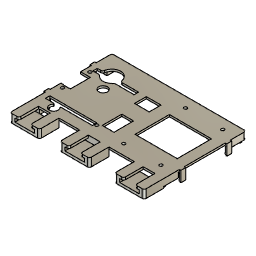
nextion_display_obd_holder_FUSION360 (Autodesk Fusion 360 design; units mm, degrees)
Autodesk Fusion 360 part; units mm, degrees
sketch "Sketch1" plane through (0, 0, 0) normal (0, 0, 1) x (1, 0, 0)
  line L0 (68.45, -42) -> (-68.45, -42)
  line L1 (-68.45, -42) -> (-68.45, 42)
  line L2 (-68.45, 42) -> (68.45, 42)
  line L3 (68.45, 42) -> (68.45, -42)
  line L4 (68.45, -42) -> (-68.45, 42) construction
  line L5 (-68.45, -42) -> (68.45, 42) construction
  line L6 (65.25, -38.9) -> (-65.25, -38.9) construction
  line L7 (-65.25, -38.9) -> (-65.25, 38.9) construction
  line L8 (-65.25, 38.9) -> (65.25, 38.9) construction
  line L9 (65.25, 38.9) -> (65.25, -38.9) construction
  line L10 (65.25, -38.9) -> (-65.25, 38.9) construction
  line L11 (-65.25, -38.9) -> (65.25, 38.9) construction
  circle A0 centre (-65.25, 38.9) radius 1.45
  circle A1 centre (65.25, 38.9) radius 1.45
  circle A2 centre (65.25, -38.9) radius 1.45
  circle A3 centre (-65.25, -38.9) radius 1.45
  line L12 (-68.45, 42) -> (-58.45, 42)
  line L13 (-58.45, 42) -> (-58.45, 27)
  line L14 (-58.45, 27) -> (-68.45, 27)
  line L15 (-68.45, 27) -> (-68.45, 42)
  line L16 (-68.45, -42) -> (-58.45, -42)
  line L17 (-58.45, -42) -> (-58.45, -27)
  line L18 (-58.45, -27) -> (-68.45, -27)
  line L19 (68.45, 42) -> (58.45, 42)
  line L20 (58.45, 42) -> (58.45, 27)
  line L21 (58.45, 27) -> (68.45, 27)
  line L22 (68.45, 27) -> (68.45, 42)
  line L23 (68.45, -42) -> (58.45, -42)
  line L24 (58.45, -42) -> (58.45, -27)
  line L25 (58.45, -27) -> (68.45, -27)
  line L26 (68.45, -27) -> (68.45, -42)
  line L27 (25, -30) -> (-25, -30)
  line L28 (-25, -30) -> (-25, 30)
  line L29 (-25, 30) -> (25, 30)
  line L30 (25, 30) -> (25, -30)
  line L31 (25, -30) -> (-25, 30) construction
  line L32 (-25, -30) -> (25, 30) construction
  line L33 (-58.45, -10) -> (-68.45, -10)
  line L34 (-68.45, -10) -> (-68.45, 10)
  line L35 (-68.45, 10) -> (-58.45, 10)
  line L36 (-58.45, 10) -> (-58.45, -10)
  line L37 (-58.45, -10) -> (-68.45, 10) construction
  line L38 (-68.45, -10) -> (-58.45, 10) construction
  line L39 (-12.45, -35) -> (7.55, -35)
  line L40 (7.55, -35) -> (7.55, -42)
  line L41 (7.55, -42) -> (-12.45, -42)
  line L42 (-12.45, -42) -> (-12.45, -35)
  circle A4 centre (-48.45, 22) radius 9
  circle A5 centre (-50.45, -35.5) radius 4.5
  circle A6 centre (-41.45, 6) radius 4.5
  line L43 (68.45, -21) -> (69.95, -21)
  line L44 (69.95, -21) -> (69.95, -26)
  line L45 (69.95, -26) -> (68.45, -26)
  line L46 (68.45, -26) -> (68.45, -21)
  point P0 (-63.45, 0)
  dimension "d1" = 136.9
  dimension "d2" = 84
  dimension "d3" = 130.5
  dimension "d4" = 77.8
  dimension "d5" = 2.9
  dimension "d6" = 2.9
  dimension "d7" = 2.9
  dimension "d8" = 2.9
  dimension "d9" = 10
  dimension "d10" = 15
  dimension "d11" = 10
  dimension "d12" = 15
  dimension "d13" = 10
  dimension "d14" = 15
  dimension "d15" = 10
  dimension "d16" = 15
  dimension "d25" = 50
  dimension "d26" = 60
  dimension "d60" = 10
  dimension "d61" = 20
  dimension "d62" = 20
  dimension "d63" = 7
  dimension "d64" = 18
  dimension "d65" = 20
  dimension "d66" = 20
  dimension "d67" = 9
  dimension "d68" = 18
  dimension "d69" = 6.5
  dimension "d70" = 9
  dimension "d71" = 27
  dimension "d72" = 36
  dimension "d134" = 56
  dimension "d148" = 1.5
  dimension "d149" = 5
  dimension "d150" = 1
  constraint horizontal L0
  constraint perpendicular L0 L1
  constraint parallel L0 L2
  constraint parallel L1 L3
  constraint coincident L4 origin
  constraint coincident L5 origin
  constraint horizontal L6
  constraint perpendicular L6 L7
  constraint parallel L6 L8
  constraint parallel L7 L9
  constraint coincident L10 origin
  constraint coincident L11 origin
  constraint coincident L7.end L8.start
  constraint coincident L8.end L9.start
  constraint coincident L6.start L9.end
  constraint coincident L6.end L7.start
  constraint horizontal L12
  constraint vertical L13
  constraint horizontal L14
  constraint vertical L15
  constraint horizontal L16
  constraint vertical L17
  constraint horizontal L18
  constraint horizontal L19
  constraint vertical L20
  constraint horizontal L21
  constraint vertical L22
  constraint horizontal L23
  constraint vertical L24
  constraint horizontal L25
  constraint vertical L26
  constraint horizontal L27
  constraint perpendicular L27 L28
  constraint parallel L27 L29
  constraint parallel L28 L30
  constraint coincident L31 origin
  constraint coincident L32 origin
  constraint horizontal L33
  constraint perpendicular L33 L34
  constraint parallel L33 L35
  constraint parallel L34 L36
  constraint coincident L37 P0
  constraint coincident L38 P0
  constraint midpoint L1 L34
  constraint horizontal L39
  constraint vertical L40
  constraint horizontal L41
  constraint vertical L42
  constraint horizontal L43
  constraint vertical L44
  constraint horizontal L45
  constraint vertical L46
  constraint coincident L3 L43.start
  measures "d1" distance of L1.end L2.end
  measures "d2" distance of L0.end L1.end
  measures "d3" distance of L7.end L8.end
  measures "d4" distance of L6.end L7.end
  measures "d5" diameter of A0
  measures "d6" diameter of A1
  measures "d7" diameter of A2
  measures "d8" diameter of A3
  measures "d9" distance of L1.end L12.end
  measures "d10" distance of L1.end L14.end
  measures "d11" distance of L0.end L16.end
  measures "d12" distance of L0.end L18.end
  measures "d13" distance of L2.end L19.end
  measures "d14" distance of L2.end L21.end
  measures "d15" distance of L0.start L23.end
  measures "d16" distance of L0.start L25.end
  measures "d25" distance of L28.end L29.end
  measures "d26" distance of L27.end L28.end
  measures "d60" distance of L34.end L35.end
  measures "d61" distance of L33.end L34.end
  measures "d62" distance of L39.start L39.end
  measures "d63" distance of L39.start L41.end
  measures "d64" diameter of A4
  measures "d65" distance of L2 A4.centre
  measures "d66" distance of L1 A4.centre
  measures "d67" diameter of A5
  measures "d68" distance of L1 A5.centre
  measures "d69" distance of L0 A5.centre
  measures "d70" diameter of A6
  measures "d71" distance of L1 A6.centre
  measures "d72" distance of L2 A6.centre
  measures "d134" distance of L1 L42
  measures "d148" distance of L43.start L43.end
  measures "d149" distance of L43.start L45.end
  measures "d150" distance of L25 L45
extrude "Extrude1" add sketch "Sketch1" along normal blind 2 contours L0 L3 L23 L24 L25 L26 | L0 L1 L2 L3 L13 L14 L17 L18 L20 L21 L24 L25 L33 L35 L36 L39 L40 L42 L46 | L0 L39 L40 L41 L42 | L0 L1 L16 L17 L18 | L2 L3 L19 L20 L21 L22 | L1 L2 L12 L13 L14 L15 | A0 | A1 | A2 | A3 | L27 L28 L29 L30 makes body 1
extrude "Extrude2" add sketch "Sketch1" against normal blind 5 contours L0 L3 L23 L24 L25 L26 | L0 L39 L40 L41 L42 | L0 L1 L16 L17 L18 | L2 L3 L19 L20 L21 L22 | L1 L2 L12 L13 L14 L15 bodies 1
extrude "Extrude3" add sketch "Sketch1" against normal blind 8 contours A0 | A1 | A2 | A3 bodies 1
chamfer "Chamfer1" distance 0.5 angle 45 4 edges at (63.8981, 39.4243, -8) (63.8981, -38.3757, -8) (-66.6019, -38.3757, -8) (-66.6019, 39.4243, -8) on bodies 1
fillet "Fillet2" radius 2 2 edges at (-68.45, 42, -1.5) (68.45, 42, -1.5) on bodies 1
sketch "Sketch6" plane through (0, 0, 2) normal (0, 0, 1) x (-1, 0, 0)
  arc A0 (-68.45, -40) -> (-66.45, -42) centre (-66.45, -40) ccw
  line L0 (-66.45, -42) -> (66.45, -42)
  arc A1 (66.45, -42) -> (68.45, -40) centre (66.45, -40) ccw
  line L1 (68.45, -40) -> (68.45, -10)
  line L2 (68.45, -10) -> (58.45, -10)
  line L3 (58.45, -10) -> (58.45, 10)
  line L4 (58.45, 10) -> (68.45, 10)
  line L5 (68.45, 10) -> (68.45, 42)
  line L6 (68.45, 42) -> (-68.45, 42)
  line L7 (-68.45, 42) -> (-68.45, -40)
  circle A2 centre (48.45, -22) radius 9
  circle A3 centre (41.45, -6) radius 4.5
  circle A4 centre (50.45, 35.5) radius 4.5
  line L8 (-60.7116, 31.6265) -> (-22.7116, 31.6265)
  line L9 (-22.7116, 31.6265) -> (-22.7116, -31.3735)
  line L10 (-22.7116, -31.3735) -> (-60.7116, -31.3735)
  line L11 (-60.7116, -31.3735) -> (-60.7116, 31.6265)
  line L12 (-60.7116, 31.6265) -> (-22.7116, -31.3735) construction
  line L13 (-22.7116, 31.6265) -> (-60.7116, -31.3735) construction
  point P0 (-41.7116, 0.1265)
  dimension "d91" = 38
  dimension "d92" = 63
  constraint horizontal L8
  constraint perpendicular L8 L9
  constraint parallel L8 L10
  constraint parallel L9 L11
  constraint coincident L12 P0
  constraint coincident L13 P0
  measures "d91" distance of L9.end L10.end
  measures "d92" distance of L8.end L9.end
sketch "Sketch7" plane through (0, 0, 0) normal (0, 0, 1) x (1, 0, 0)
  line L0 (55.2284, -31.5) -> (17.2284, -31.5)
  line L1 (17.2284, -31.5) -> (17.2284, 31.5)
  line L2 (17.2284, 31.5) -> (55.2284, 31.5)
  line L3 (55.2284, 31.5) -> (55.2284, -31.5)
  line L4 (55.2284, -31.5) -> (17.2284, 31.5) construction
  line L5 (17.2284, -31.5) -> (55.2284, 31.5) construction
  line L6 (57.7284, -17.5) -> (14.7284, -17.5)
  line L7 (14.7284, -17.5) -> (14.7284, 17.5)
  line L8 (14.7284, 17.5) -> (57.7284, 17.5)
  line L9 (57.7284, 17.5) -> (57.7284, -17.5)
  line L10 (57.7284, -17.5) -> (14.7284, 17.5) construction
  line L11 (14.7284, -17.5) -> (57.7284, 17.5) construction
  point P0 (36.2284, 0)
  point P1 (36.2284, 0)
  dimension "d95" = 38
  dimension "d96" = 63
  dimension "d97" = 43
  dimension "d98" = 35
  dimension "d135" = 31.5
  constraint horizontal L0
  constraint perpendicular L0 L1
  constraint parallel L0 L2
  constraint parallel L1 L3
  constraint coincident L4 P1
  constraint coincident L5 P1
  constraint horizontal L6
  constraint perpendicular L6 L7
  constraint parallel L6 L8
  constraint parallel L7 L9
  constraint coincident L10 P1
  constraint coincident L11 P1
  constraint coincident P1 P0
  measures "d95" distance of L1.end L2.end
  measures "d96" distance of L0.end L1.end
  measures "d97" distance of L7.end L8.end
  measures "d98" distance of L6.end L7.end
  measures "d135" distance of origin L2
hole "Hole1" at (17.2284, 31.5, 0) at (55.2284, 31.5, 0) at (55.2284, -31.5, 0) at (17.2284, -31.5, 0) direction (0, 0, 1) diameter 3.2 depth 26 tip angle 180 bodies 1
extrude "Extrude8" cut sketch "Sketch7" along normal blind 19 contours L1 L3 L6 L8 | L3 L6 L8 L9 | L1 L6 L7 L8 bodies 1
sketch "Sketch8" plane through (0, 0, 0) normal (0, 0, 1) x (1, 0, 0)
  line L0 (2.0938, 21.5699) -> (-62.9062, 21.5699)
  line L1 (2.0938, 21.5699) -> (2.0938, -31.4301)
  line L2 (-62.9062, 21.5699) -> (-62.9062, 19.5699)
  line L3 (-62.9062, 19.5699) -> (-62.9062, 16.5699) construction
  line L4 (-62.9062, 16.5699) -> (-65.9062, 16.5699) construction
  line L5 (2.0938, -31.4301) -> (-62.9062, -31.4301)
  line L6 (-62.9062, -31.4301) -> (-62.9062, -18.4301)
  line L7 (-62.9062, -18.4301) -> (-62.9062, -15.4301) construction
  line L8 (-62.9062, -15.4301) -> (-65.9062, -15.4301) construction
  line L9 (-62.9062, -18.4301) -> (-65.9062, -15.4301)
  line L10 (-65.9062, -15.4301) -> (-65.9062, 16.5699)
  line L11 (-65.9062, 16.5699) -> (-62.9062, 19.5699)
  circle A0 centre (-12.9062, -28.9301) radius 1.6
  circle A1 centre (-63.4062, 14.5699) radius 1.6
  circle A2 centre (-63.4062, -13.4301) radius 1.6
  line L12 (2.0938, 21.5699) -> (-12.9062, 21.5699)
  line L13 (-12.9062, 21.5699) -> (-12.9062, 9.5699)
  line L14 (-12.9062, 9.5699) -> (2.0938, 9.5699)
  line L15 (2.0938, 9.5699) -> (2.0938, 21.5699)
  line L16 (2.0938, -6.4301) -> (-9.9062, -6.4301)
  line L17 (-9.9062, -6.4301) -> (-9.9062, -26.4301)
  line L18 (-9.9062, -26.4301) -> (2.0938, -26.4301)
  line L19 (2.0938, -26.4301) -> (2.0938, -6.4301)
  line L20 (-62.9062, 21.5699) -> (-20.9062, 21.5699)
  line L21 (-20.9062, 21.5699) -> (-20.9062, 17.0699)
  line L22 (-20.9062, 17.0699) -> (-62.9062, 17.0699)
  line L23 (-62.9062, 17.0699) -> (-62.9062, 21.5699)
  line L24 (-62.9062, -31.4301) -> (-14.9062, -31.4301)
  line L25 (-14.9062, -31.4301) -> (-14.9062, -26.9301)
  line L26 (-14.9062, -26.9301) -> (-62.9062, -26.9301)
  line L27 (-62.9062, -26.9301) -> (-62.9062, -31.4301)
  line L28 (-65.9062, -1.4301) -> (-59.9062, -1.4301)
  line L29 (-59.9062, -1.4301) -> (-59.9062, -10.4301)
  line L30 (-59.9062, -10.4301) -> (-65.9062, -10.4301)
  line L31 (-65.9062, -10.4301) -> (-65.9062, -1.4301)
  dimension "d104" = 65
  dimension "d105" = 53
  dimension "d106" = 2
  dimension "d107" = 3
  dimension "d108" = 3
  dimension "d109" = 65
  dimension "d110" = 13
  dimension "d111" = 3
  dimension "d112" = 3
  dimension "d113" = 3.2
  dimension "d114" = 15
  dimension "d115" = 50.5
  dimension "d116" = 3.2
  dimension "d117" = 65.5
  dimension "d118" = 3.2
  dimension "d119" = 65.5
  dimension "d120" = 7
  dimension "d121" = 35
  dimension "d122" = 15
  dimension "d123" = 12
  dimension "d124" = 12
  dimension "d125" = 20
  dimension "d126" = 5
  dimension "d136" = 42
  dimension "d137" = 4.5
  dimension "d138" = 48
  dimension "d139" = 4.5
  dimension "d140" = 6
  dimension "d141" = 9
  dimension "d142" = 21
  constraint perpendicular L0 L1
  constraint perpendicular L0 L2
  constraint parallel L2 L3
  constraint perpendicular L3 L4
  constraint perpendicular L1 L5
  constraint perpendicular L5 L6
  constraint parallel L6 L7
  constraint perpendicular L7 L8
  constraint horizontal L12
  constraint vertical L13
  constraint horizontal L14
  constraint vertical L15
  constraint horizontal L16
  constraint vertical L17
  constraint horizontal L18
  constraint vertical L19
  constraint coincident L1 L16.start
  constraint horizontal L20
  constraint vertical L21
  constraint horizontal L22
  constraint vertical L23
  constraint horizontal L24
  constraint vertical L25
  constraint horizontal L26
  constraint vertical L27
  constraint horizontal L28
  constraint vertical L29
  constraint horizontal L30
  constraint vertical L31
  constraint coincident L10 L28.start
  measures "d104" distance of L0.start L0.end
  measures "d105" distance of L0.start L1.end
  measures "d106" distance of L0.end L2.end
  measures "d107" distance of L2.end L3.end
  measures "d108" distance of L3.end L4.end
  measures "d109" distance of L1.end L5.end
  measures "d110" distance of L5.end L6.end
  measures "d111" distance of L6.end L7.end
  measures "d112" distance of L7.end L8.end
  measures "d113" diameter of A0
  measures "d114" distance of L1 A0.centre
  measures "d115" distance of L0 A0.centre
  measures "d116" diameter of A1
  measures "d117" distance of L1 A1.centre
  measures "d118" diameter of A2
  measures "d119" distance of L1 A2.centre
  measures "d120" distance of L0 A1.centre
  measures "d121" distance of L0 A2.centre
  measures "d122" distance of L0.start L12.end
  measures "d123" distance of L0.start L14.end
  measures "d124" distance of L16.start L16.end
  measures "d125" distance of L16.start L18.end
  measures "d126" distance of L5 L18
  measures "d136" distance of L0.end L20.end
  measures "d137" distance of L0.end L22.end
  measures "d138" distance of L5.end L24.end
  measures "d139" distance of L5.end L26.end
  measures "d140" distance of L28.start L28.end
  measures "d141" distance of L28.start L30.end
  measures "d142" distance of L5 L30
extrude "Extrude9" cut sketch "Sketch8" along normal blind 10 contours L0 L1 L12 L13 L14 L15 | L1 L16 L17 L18 L19 bodies 1
extrude "Extrude10" cut sketch "Sketch8" along normal blind 5 contours A0 | A1 | A2 bodies 1
sketch "Sketch9" plane through (0, 0, 0) normal (0, 0, -1) x (1, 0, 0)
  circle A0 centre (-63.4062, -14.5699) radius 1.6
  circle A1 centre (-63.4062, 13.4301) radius 1.6
  circle A2 centre (-12.9062, 28.9301) radius 1.6
  line L0 (-12.9062, -9.5699) -> (2.0938, -9.5699)
  line L1 (2.0938, -9.5699) -> (2.0938, -21.5699)
  line L2 (2.0938, -21.5699) -> (-12.9062, -21.5699)
  line L3 (-12.9062, -21.5699) -> (-12.9062, -9.5699)
  line L4 (-9.9062, 26.4301) -> (2.0938, 26.4301)
  line L5 (2.0938, 26.4301) -> (2.0938, 6.4301)
  line L6 (2.0938, 6.4301) -> (-9.9062, 6.4301)
  line L7 (-9.9062, 6.4301) -> (-9.9062, 26.4301)
  line L8 (57.7284, 17.5) -> (57.7284, -17.5)
  line L9 (57.7284, -17.5) -> (14.7284, -17.5)
  line L10 (14.7284, -17.5) -> (14.7284, 17.5)
  line L11 (14.7284, 17.5) -> (57.7284, 17.5)
  circle A3 centre (55.2284, 31.5) radius 1.6
  circle A4 centre (17.2284, -31.5) radius 1.6
  circle A5 centre (55.2284, -31.5) radius 1.6
  circle A6 centre (17.2284, 31.5) radius 1.6
  line L12 (-12.45, 35) -> (-12.45, 42)
  line L13 (-12.45, 42) -> (-58.45, 42)
  line L14 (-58.45, 42) -> (-58.45, 27)
  line L15 (-58.45, 27) -> (-68.45, 27)
  line L16 (-68.45, 10) -> (-58.45, 10)
  line L17 (-58.45, 10) -> (-58.45, -10)
  line L18 (-58.45, -10) -> (-68.45, -10)
  line L19 (-68.45, -27) -> (-58.45, -27)
  line L20 (-58.45, -27) -> (-58.45, -42)
  line L21 (-58.45, -42) -> (58.45, -42)
  line L22 (58.45, -42) -> (58.45, -27)
  line L23 (58.45, -27) -> (68.45, -27)
  line L24 (68.45, 27) -> (58.45, 27)
  line L25 (58.45, 27) -> (58.45, 42)
  line L26 (58.45, 42) -> (7.55, 42)
  line L27 (7.55, 42) -> (7.55, 35)
  line L28 (7.55, 35) -> (-12.45, 35)
  circle A7 centre (-48.45, -22) radius 9
  circle A8 centre (-41.45, -6) radius 4.5
  circle A9 centre (-50.45, 35.5) radius 4.5
  line L29 (-58.45, -42) -> (58.45, -42)
  line L30 (58.45, -42) -> (58.45, -39)
  line L31 (58.45, -39) -> (-58.45, -39)
  line L32 (-58.45, -39) -> (-58.45, -42)
  line L33 (-68.45, 27) -> (-68.45, 10)
  line L34 (-68.45, -10) -> (-68.45, -27)
  line L35 (68.45, -27) -> (68.45, 27)
  dimension "d131" = 3
  constraint horizontal L29
  constraint vertical L30
  constraint horizontal L31
  constraint vertical L32
  constraint coincident L20.end L21.start
  measures "d131" distance of L20.end L31.end
extrude "Extrude11" add sketch "Sketch9" along normal blind 2 contours L20 L21 L22 L29 L30 L31 L32 bodies 1
extrude "Extrude12" cut sketch "Sketch8" along normal blind 10 contours L0 L2 L20 L21 L22 L23 | L5 L6 L24 L25 L26 L27 | L10 L28 L29 L30 L31 bodies 1
sketch "Sketch10" plane through (0, -42, 0) normal (0, -1, 0) x (1, 0, 0)
  line L0 (58.45, -5) -> (68.45, -5)
  line L1 (-58.45, -5) -> (-58.45, 0)
  line L2 (-58.45, 0) -> (-12.45, 0)
  line L3 (-12.45, 0) -> (-12.45, -5)
  line L4 (-12.45, -5) -> (7.55, -5)
  line L5 (7.55, -5) -> (7.55, 0)
  line L6 (7.55, 0) -> (58.45, 0)
  line L7 (58.45, 0) -> (58.45, -5)
  line L8 (68.45, 2) -> (-68.45, 2)
  line L9 (-12.45, 0) -> (-12.45, 2)
  line L10 (7.55, 0) -> (7.55, 2)
  line L11 (68.45, -5) -> (68.45, 2)
  line L12 (-68.45, 2) -> (-68.45, -5)
  line L13 (-68.45, -5) -> (-58.45, -5)
  constraint coincident L2.end L3.start
  constraint coincident L8 L9.end
  constraint perpendicular L8 L9
  constraint coincident L5.end L6.start
  constraint coincident L8 L10.end
  constraint perpendicular L8 L10
extrude "Extrude13" add sketch "Sketch10" along normal blind 20 contours L3 L4 L5 L8 L9 L10 bodies 1
chamfer "Chamfer2" [suppressed]
sketch "Sketch2" plane through (0, 0, 0) normal (0, 0, 1) x (1, 0, 0)
  line L0 (68.45, -42) -> (-68.45, -42)
  line L1 (-68.45, -42) -> (-68.45, 42)
  line L2 (-68.45, 42) -> (68.45, 42)
  line L3 (68.45, 42) -> (68.45, -42)
  line L4 (68.45, -42) -> (-68.45, 42) construction
  line L5 (-68.45, -42) -> (68.45, 42) construction
  line L6 (-171.1068, -19.3221) -> (-106.1068, -19.3221)
  line L7 (-106.1068, -19.3221) -> (-106.1068, -17.3221)
  line L8 (-171.1068, -19.3221) -> (-171.1068, 33.6779)
  line L9 (-171.1068, 33.6779) -> (-106.1068, 33.6779)
  line L10 (-106.1068, 33.6779) -> (-106.1068, 20.6779)
  line L11 (-106.1068, 20.6779) -> (-106.1068, 17.6779) construction
  line L12 (-106.1068, -17.3221) -> (-106.1068, -14.3221) construction
  line L13 (-106.1068, 17.6779) -> (-103.1068, 17.6779) construction
  line L14 (-106.1068, -14.3221) -> (-103.1068, -14.3221) construction
  line L15 (-106.1068, -17.3221) -> (-103.1068, -14.3221)
  line L16 (-106.1068, 20.6779) -> (-103.1068, 17.6779)
  line L17 (-103.1068, 17.6779) -> (-103.1068, -14.3221)
  circle A0 centre (-156.1068, 31.1779) radius 1.6
  circle A1 centre (-105.6068, -12.3221) radius 1.6
  circle A2 centre (-105.6068, 15.6779) radius 1.6
  line L18 (-134.6413, -60.8308) -> (-91.6413, -60.8308)
  line L19 (-91.6413, -60.8308) -> (-91.6413, -130.0308)
  line L20 (-91.6413, -130.0308) -> (-134.6413, -130.0308)
  line L21 (-134.6413, -130.0308) -> (-134.6413, -60.8308)
  dimension "d38" = 136.9
  dimension "d39" = 84
  dimension "d40" = 65
  dimension "d41" = 2
  dimension "d42" = 53
  dimension "d43" = 65
  dimension "d44" = 13
  dimension "d45" = 3
  dimension "d46" = 3
  dimension "d47" = 3
  dimension "d48" = 3
  dimension "d49" = 3.2
  dimension "d50" = 15
  dimension "d51" = 50.5
  dimension "d52" = 3.2
  dimension "d53" = 65.5
  dimension "d54" = 7
  dimension "d55" = 3.2
  dimension "d56" = 35
  dimension "d57" = 65.5
  dimension "d58" = 43
  dimension "d59" = 69.2
  constraint horizontal L0
  constraint perpendicular L0 L1
  constraint parallel L0 L2
  constraint parallel L1 L3
  constraint coincident L4 origin
  constraint coincident L5 origin
  constraint horizontal L6
  constraint perpendicular L6 L7
  constraint perpendicular L6 L8
  constraint perpendicular L8 L9
  constraint perpendicular L9 L10
  constraint parallel L10 L11
  constraint parallel L7 L12
  constraint perpendicular L11 L13
  constraint perpendicular L12 L14
  constraint horizontal L18
  constraint vertical L19
  constraint horizontal L20
  constraint vertical L21
  measures "d38" distance of L1.end L2.end
  measures "d39" distance of L0.end L1.end
  measures "d40" distance of L6.start L6.end
  measures "d41" distance of L6.end L7.end
  measures "d42" distance of L6.start L8.end
  measures "d43" distance of L8.end L9.end
  measures "d44" distance of L9.end L10.end
  measures "d45" distance of L10.end L11.end
  measures "d46" distance of L7.end L12.end
  measures "d47" distance of L11.end L13.end
  measures "d48" distance of L12.end L14.end
  measures "d49" diameter of A0
  measures "d50" distance of L8 A0.centre
  measures "d51" distance of L6 A0.centre
  measures "d52" diameter of A1
  measures "d53" distance of L8 A1.centre
  measures "d54" distance of L6 A1.centre
  measures "d55" diameter of A2
  measures "d56" distance of L6 A2.centre
  measures "d57" distance of L8 A2.centre
  measures "d58" distance of L18.start L18.end
  measures "d59" distance of L18.start L20.end
extrude "Extrude14" add sketch "Sketch1" along normal blind 2 separate body contours L3 L43 L44 L45 L46 makes body 2
extrude "Extrude15" add sketch "Sketch1" against normal blind 9 contours L3 L43 L44 L45 L46 bodies 2
sketch "Sketch11" plane through (0, -26, 0) normal (0, -1, 0) x (1, 0, 0)
  line L0 (69.95, -9) -> (69.95, 2)
  line L1 (69.95, 2) -> (68.45, 2)
  line L2 (68.45, 2) -> (68.45, -9)
  line L3 (68.45, -9) -> (69.95, -9)
  line L4 (68.45, 2) -> (68.45, -5)
  line L5 (68.45, -5) -> (68.45, -6.6)
  line L6 (68.45, -6.6) -> (67.7429, -7.3071)
  line L7 (68.45, -6.6) -> (69.45, -6.6) construction
  line L8 (67.7429, -7.3071) -> (70.1365, -9.7007)
  line L9 (67.7429, -7.3071) -> (70.7602, -7.3071) construction
  dimension "d155" = 7
  dimension "d156" = 1.6
  dimension "d157" = 135
  dimension "d158" = 1
  dimension "d159" = 45
  constraint coincident L1.end L2.start
  constraint perpendicular L1 L4
  constraint parallel L2 L5
  constraint horizontal L7
  constraint horizontal L9
  measures "d155" distance of L1.end L4.end
  measures "d156" distance of L4.end L5.end
  measures "d157" angle of L6 L7
  measures "d158" distance of L5.end L6.end
  measures "d159" angle of L8 L9
extrude "Extrude16" add sketch "Sketch11" against normal blind 5 contours L2 L6 L8 bodies 2
extrude "Extrude17" cut sketch "Sketch11" against normal blind 5 contours L2 L3 L8 bodies 2
mirror "Mirror1" about plane through (0, 0, 0) normal (0, 1, 0) of bodies 2 makes body 3
mirror "Mirror2" about plane through (0, 0, 0) normal (1, 0, 0) of bodies 3 2 makes body 4 at (-69.95, -22.6667, -5.3333) makes body 5 at (-69.95, 22.6667, -5.3333)
combine "Combine1" operation add target body 1 tool bodies 2 3 4 5
chamfer "Chamfer4" distance 1 angle 45 4 edges at (68.45, 23.5, 0) (68.45, -23.5, 0) (-68.45, 23.5, 0) (-68.45, -23.5, 0) on bodies 1
fillet "Fillet3" radius 0.5 2 edges at (-48.5301, -31.4301, 1) (-52.3699, -31.4301, 1) on bodies 1
extrude "Extrude18" cut 1 faces at (-61.4208, -28.4767, 0) along direction (0, 0, -1) blind 5 on bodies 1 bodies 1
fillet "Fillet4" radius 2 4 edges at (-40.9205, 17.0699, 1) (-55.9795, 17.0699, 1) (-57.4397, 21.5699, 1) (-39.4603, 21.5699, 1) on bodies 1
sketch "Sketch12" plane through (0, -62, 0) normal (0, -1, 0) x (1, 0, 0)
  line L0 (-12.45, 2) -> (-12.45, -5)
  line L1 (-12.45, -5) -> (7.55, -5)
  line L2 (7.55, -5) -> (7.55, 2)
  line L3 (7.55, 2) -> (-12.45, 2)
  line L4 (-8.45, 2) -> (3.55, 2)
  line L5 (3.55, 2) -> (3.55, -0.5)
  line L6 (3.55, -0.5) -> (-8.45, -0.5)
  line L7 (-8.45, -0.5) -> (-8.45, 2)
  line L8 (-12.45, -0.5) -> (7.55, -0.5)
  line L9 (7.55, -0.5) -> (7.55, -4)
  line L10 (7.55, -4) -> (-12.45, -4)
  line L11 (-12.45, -4) -> (-12.45, -0.5)
  line L12 (7.55, 2) -> (12.55, 2)
  line L13 (12.55, 2) -> (12.55, -5)
  line L14 (12.55, -5) -> (7.55, -5)
  line L15 (7.55, -5) -> (7.55, 2)
  line L16 (-12.45, 2) -> (-17.45, 2)
  line L17 (-17.45, 2) -> (-17.45, -5)
  line L18 (-17.45, -5) -> (-12.45, -5)
  line L19 (-12.45, -5) -> (-12.45, 2)
  line L20 (-8.45, -0.5) -> (-8.45, 1.5)
  line L21 (-8.45, 1.5) -> (-10.8867, -0.9367)
  line L22 (-8.45, 1.5) -> (-5.3575, 1.5) construction
  line L23 (3.55, -0.5) -> (3.55, 1.5)
  line L24 (3.55, 1.5) -> (5.9561, -0.9061)
  line L25 (3.55, 1.5) -> (6.5991, 1.5) construction
  dimension "d176" = 12
  dimension "d177" = 2.5
  dimension "d178" = 20
  dimension "d179" = 3.5
  dimension "d180" = 5
  dimension "d181" = 5
  dimension "d184" = 2
  dimension "d185" = 135
  dimension "d186" = 2
  dimension "d187" = 45
  constraint horizontal L4
  constraint vertical L5
  constraint horizontal L6
  constraint vertical L7
  constraint midpoint L3 L4
  constraint horizontal L8
  constraint vertical L9
  constraint horizontal L10
  constraint vertical L11
  constraint midpoint L6 L8
  constraint horizontal L12
  constraint vertical L13
  constraint horizontal L14
  constraint vertical L15
  constraint coincident L2.end L3.start
  constraint horizontal L16
  constraint vertical L17
  constraint horizontal L18
  constraint vertical L19
  constraint coincident L0.start L3.end
  constraint perpendicular L8 L20
  constraint horizontal L22
  constraint perpendicular L8 L23
  constraint horizontal L25
  measures "d176" distance of L4.start L4.end
  measures "d177" distance of L4.start L6.end
  measures "d178" distance of L8.start L8.end
  measures "d179" distance of L8.start L10.end
  measures "d180" distance of L2.end L12.end
  measures "d181" distance of L0.start L16.end
  measures "d184" distance of L6.end L20.end
  measures "d185" angle of L21 L22
  measures "d186" distance of L5.end L23.end
  measures "d187" angle of L24 L25
extrude "Extrude19" add sketch "Sketch12" against normal blind 20 contours L0 L11 L16 L17 L18 L19 | L2 L9 L12 L13 L14 L15 bodies 1
extrude "Extrude20" cut sketch "Sketch12" against normal blind 20 contours L0 L2 L6 L8 L9 L10 L11 L15 L19 | L3 L4 L5 L6 L7 L8 L20 L23 bodies 1
fillet "Fillet5" radius 2 2 edges at (-8.45, -62, 0.75) (3.55, -62, 0.75) on bodies 1
fillet "Fillet6" radius 2 2 edges at (12.55, -62, -1.5) (-17.45, -62, -1.5) on bodies 1
sketch "Sketch13" plane through (0, 0, -5) normal (0, 0, -1) x (1, 0, 0)
  arc A0 (-15.45, 62) -> (-17.45, 60) centre (-15.45, 60) ccw
  line L0 (-17.45, 60) -> (-17.45, 42)
  line L1 (-17.45, 42) -> (-12.45, 42)
  line L2 (-12.45, 42) -> (-12.45, 35)
  line L3 (-12.45, 35) -> (7.55, 35)
  line L4 (7.55, 35) -> (7.55, 42)
  line L5 (7.55, 42) -> (12.55, 42)
  line L6 (12.55, 42) -> (12.55, 60)
  arc A1 (12.55, 60) -> (10.55, 62) centre (10.55, 60) ccw
  line L7 (10.55, 62) -> (-15.45, 62)
  line L8 (7.55, 42) -> (-12.45, 42)
  constraint coincident L4.end L5.start
  constraint coincident L1.end L2.start
extrude "Extrude21" add sketch "Sketch13" along normal blind 1.6 contours A0 L0 L1 L5 L6 A1 L7 L8 bodies 1
sketch "Sketch14" plane through (0, -42, 0) normal (0, -1, 0) x (1, 0, 0)
  line L0 (-17.45, 0) -> (-17.45, 2)
  line L1 (-17.45, 2) -> (-68.45, 2)
  line L2 (-68.45, 2) -> (-68.45, -5)
  line L3 (-68.45, -5) -> (-58.45, -5)
  line L4 (-58.45, -5) -> (-58.45, 0)
  line L5 (-58.45, 0) -> (-17.45, 0)
  line L6 (-68.45, 2) -> (-63.45, 2)
  line L7 (-63.45, 2) -> (-63.45, -0.5)
  line L8 (-63.45, -0.5) -> (-68.45, -0.5)
  line L9 (-68.45, -0.5) -> (-68.45, 2)
  line L10 (-63.45, 2) -> (-43.45, 2)
  line L11 (-43.45, 2) -> (-43.45, -0.5)
  line L12 (-43.45, -0.5) -> (-63.45, -0.5)
  line L13 (-63.45, -0.5) -> (-63.45, 2)
  line L14 (-43.45, 2) -> (-38.45, 2)
  line L15 (-38.45, 2) -> (-38.45, -0.5)
  line L16 (-38.45, -0.5) -> (-43.45, -0.5)
  line L17 (-43.45, -0.5) -> (-43.45, 2)
  line L18 (-68.45, -0.5) -> (-38.45, -0.5)
  line L19 (-38.45, -0.5) -> (-38.45, -4)
  line L20 (-38.45, -4) -> (-68.45, -4)
  line L21 (-68.45, -4) -> (-68.45, -0.5)
  line L22 (-68.45, -4) -> (-38.45, -4)
  line L23 (-38.45, -4) -> (-38.45, -6.6)
  line L24 (-38.45, -6.6) -> (-68.45, -6.6)
  line L25 (-68.45, -6.6) -> (-68.45, -4)
  line L26 (-59.45, 2) -> (-47.45, 2)
  line L27 (-47.45, 2) -> (-47.45, -0.5)
  line L28 (-47.45, -0.5) -> (-59.45, -0.5)
  line L29 (-59.45, -0.5) -> (-59.45, 2)
  line L30 (-63.45, -0.5) -> (-63.45, -4)
  line L31 (-43.45, -0.5) -> (-43.45, -4)
  dimension "d196" = 5
  dimension "d197" = 2.5
  dimension "d198" = 20
  dimension "d199" = 2.5
  dimension "d200" = 5
  dimension "d201" = 2.5
  dimension "d202" = 30
  dimension "d203" = 3.5
  dimension "d204" = 30
  dimension "d205" = 2.6
  dimension "d206" = 12
  dimension "d207" = 2.5
  constraint horizontal L6
  constraint vertical L7
  constraint horizontal L8
  constraint vertical L9
  constraint coincident L1.end L2.start
  constraint horizontal L10
  constraint vertical L11
  constraint horizontal L12
  constraint vertical L13
  constraint horizontal L14
  constraint vertical L15
  constraint horizontal L16
  constraint vertical L17
  constraint horizontal L18
  constraint vertical L19
  constraint horizontal L20
  constraint vertical L21
  constraint horizontal L22
  constraint vertical L23
  constraint horizontal L24
  constraint vertical L25
  constraint horizontal L26
  constraint vertical L27
  constraint horizontal L28
  constraint vertical L29
  constraint midpoint L10 L26
  constraint coincident L22 L30.end
  constraint perpendicular L22 L30
  constraint coincident L22 L31.end
  constraint perpendicular L22 L31
  measures "d196" distance of L1.end L6.end
  measures "d197" distance of L1.end L8.end
  measures "d198" distance of L6.end L10.end
  measures "d199" distance of L6.end L7.end
  measures "d200" distance of L10.end L14.end
  measures "d201" distance of L10.end L11.end
  measures "d202" distance of L8.end L15.end
  measures "d203" distance of L8.end L20.end
  measures "d204" distance of L20.end L19.end
  measures "d205" distance of L20.end L24.end
  measures "d206" distance of L26.start L26.end
  measures "d207" distance of L26.start L28.end
extrude "Extrude22" add sketch "Sketch14" along normal blind 20 separate body contours L5 L11 L15 L16 L17 L18 | L1 L5 L11 L14 L15 L17 | L5 L11 L12 L17 L18 L27 | L1 L5 L10 L11 L17 L27 | L16 L18 L19 L20 L22 L31 | L3 L4 L20 L22 L23 L24 L25 | L1 L7 L10 L12 L13 L18 L29 | L2 L3 L4 L20 L22 L25 | L1 L2 L6 L7 L8 L9 L13 L18 | L2 L8 L18 L20 L21 L22 L30 makes body 6
fillet "Fillet7" radius 2 4 edges at (-59.45, -62, 0.75) (-47.45, -62, 0.75) (-38.45, -62, -2.3) (-68.45, -62, -2.3) on bodies 6
mirror "Mirror3" about plane through (0, 0, 0) normal (1, 0, 0) of bodies 6 makes body 7
combine "Combine2" operation add target body 1 tool bodies 6 7
equation "d135 = d96 / 2"
named bodies: "nextion_obd_holder"
